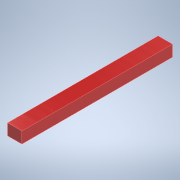
# Autodesk Inventor part: Alcance dos Sensores
Saved by Autodesk Inventor 2021 (Build 250183000, 183)
## iProperties
Created: 2022-11-17
Part Number: Alcance dos Sensores
Material: Genérico
Document SubType Name: Modeling
Designer: nicho
Surface Area: 141.7 cm^2
Volume: 57 cm^3
Appearance: Vermelho
Author: nicho
Autodesk Inventor part; units mm, degrees
ref_plane "YZ Plane" through (0, 0, 0) normal (1, 0, 0) x (0, 1, 0)
ref_plane "XZ Plane" through (0, 0, 0) normal (0, 1, 0) x (-1, 0, 0)
ref_plane "XY Plane" through (0, 0, 0) normal (0, 0, 1) x (1, 0, 0)
sketch "Esboço1" plane through (0, 0, 0) normal (0, 0, 1) x (1, 0, 0)
  line L0 (9.5, -7.5) -> (-9.5, -7.5)
  line L1 (-9.5, -7.5) -> (-9.5, 7.5)
  line L2 (-9.5, 7.5) -> (9.5, 7.5)
  line L3 (9.5, 7.5) -> (9.5, -7.5)
  line L4 (9.5, -7.5) -> (-9.5, 7.5) construction
  line L5 (-9.5, -7.5) -> (9.5, 7.5) construction
  point P0 (0, 0)
  dimension "d0" = 19
  dimension "d1" = 15
  constraints: 12 end point, 2 midpoint, 2 parallel, 1 horizontal, 1 perpendicular
  measures "d0" distance of L1.end L2.end
  measures "d1" distance of L0.end L1.end
extrude "Extrusão1" add sketch "Esboço1" along normal blind 200
